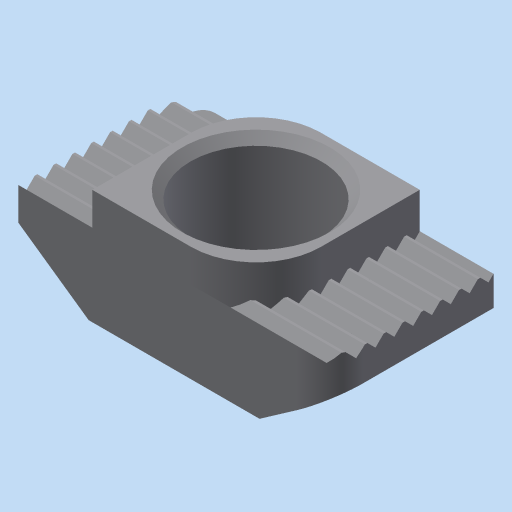
# Autodesk Inventor part: T-NUT - DropIn 4040 SERIES - M8
Saved by Autodesk Inventor 2023.2 (Build 272271000, 271)
## iProperties
Company: TraceParts S.A.
Created: 2023-02-26
Part Number: T-NUT - DropIn 4040 SERIES - M8
Checked By: TraceParts S.A.
Material: Generisch
Catalog Web Link: www.traceparts.com
Document SubType Name: Modeling
Designer: TraceParts
Density: 1 g/cm^3
Appearance: Vorgabe
REFERENCE: 07090-1008017
SUPPLIER: norelem
DESIGN: T-NUT FOR T-SLOT M08 STEEL
TraceParts.PartNumber: 30-06122017-106144
TraceParts.PartTitle: T-NUT FOR T-SLOT M08 STEEL
TraceParts.InstanceId: 30-06122017-1061443DYOD00EO1IYUO4TDSMY561GW
TRACEPARTS: TRACEPARTS
TraceParts.PartLanguage: en
TraceParts.PartVersion: 1.0.7
Author: TraceParts
Autodesk Inventor part; units mm, degrees
ref_plane "YZ Plane" through (0, 0, 0) normal (1, 0, 0) x (0, 1, 0)
ref_plane "XZ Plane" through (0, 0, 0) normal (0, 1, 0) x (-1, 0, 0)
ref_plane "XY Plane" through (0, 0, 0) normal (0, 0, 1) x (1, 0, 0)
sketch "Skizze3" plane through (0, 0, 0) normal (0, 0, 1) x (1, 0, 0)
  line L0 (0, 0) -> (5.215556, 0)
  line L1 (5.215556, 0) -> (9.5, 3)
  line L2 (9.5, 3) -> (9.5, 5)
  line L3 (9.5, 5) -> (0, 5)
  line L4 (0, 6) -> (0, -1) construction
  line L5 (0, 0) -> (-5.215556, 0)
  line L6 (-5.215556, 0) -> (-9.5, 3)
  line L7 (-9.5, 3) -> (-9.5, 5)
  line L8 (-9.5, 5) -> (0, 5)
  dimension "d6" = 9.5
  dimension "d8" = 5
  dimension "d9" = 3
  dimension "d10" = 145
  constraints: 16 end point, 3 symmetric about line, 2 perpendicular, 1 horizontal
  measures "d6" distance between parallel lines of L4 L2
  measures "d8" distance between parallel lines of L0 L3
  measures "d9" distance from line of L0 L1.end
  measures "d10" angle of L0 L1
extrude "Extrusion2" add sketch "Skizze3" along normal mid plane 10
sketch "Skizze4" plane through (-9.5, 5, 5) normal (0, 1, 0) x (1, 0, 0)
  line L0 (0, 10) -> (0, 0)
  line L1 (19, 0) -> (0, 0)
  line L2 (19, 10) -> (19, 0)
  line L3 (0, 10) -> (19, 10)
  circle A0 centre (9.5, 5) radius 4
  line L4 (4.5, 10) -> (14.5, 10)
  line L5 (14.5, 10) -> (14.5, 0)
  line L6 (14.5, 0) -> (4.5, 0)
  line L7 (4.5, 0) -> (4.5, 10)
  line L8 (4.5, 10) -> (14.5, 0) construction
  line L9 (14.5, 10) -> (4.5, 0) construction
  line L10 (0, 10) -> (19, 10)
  arc A1 (8.5, 10) -> (4.5, 6) centre (8.464449, 6.035551) ccw
  arc A2 (10.5, 0) -> (14.5, 4) centre (10.535551, 3.964449) ccw
  point P0 (4.5, 0)
  point P1 (14.5, 0)
  point P2 (4.5, 10)
  point P3 (10.571102, 0)
  point P4 (14.5, 4)
  point P5 (8.428898, 10)
  point P6 (4.5, 6.071102)
  dimension "d13" = 8
  dimension "d14" = 10
  dimension "d15" = 10
  dimension "d37" = 4
  dimension "d38" = 4
  constraints: 12 end point, 4 point on circle, 3 centre point, 3 symmetric about line, 2 midpoint, 2 parallel, 2 point on line, 1 coincident, 1 horizontal, 1 perpendicular, 1 other
  measures "d13" diameter of A0
  measures "d14" distance of L5.end L6.end
  measures "d15" distance of L4.end L5.end
  measures "d37" distance from line of L7 A1.start
  measures "d38" distance from line of L3 A1.end
sketch "Skizze4 outline for Extrusion3" plane through (-9.5, 5, 5) normal (0, 1, 0) x (1, 0, 0)
  arc A0 (10.571102, 0) -> (14.5, 4) centre (10.535551, 3.964449) ccw
  line L0 (4.5, 0) -> (10.571102, 0)
  line L1 (14.5, 4) -> (14.5, 10)
  line L2 (4.5, 6.071102) -> (4.5, 0)
  line L3 (14.5, 10) -> (8.428898, 10)
  arc A1 (8.428898, 10) -> (4.5, 6.071102) centre (8.464449, 6.035551) ccw
  circle A2 centre (9.5, 5) radius 4
extrude "Extrusion3" add sketch "Skizze4 outline for Extrusion3" along normal blind 2 and the other way blind 5 separate body
sketch "Skizze5" plane through (9.5, 3, 5) normal (1, 0, 0) x (0, 0, -1)
  line L0 (10, 2) -> (0, 2)
  line L1 (0, 0) -> (0, 2)
  line L2 (10, 0) -> (0, 0)
  line L3 (10, 2) -> (10, 0)
  line L4 (0, 0) -> (0, 2)
  line L5 (0, 2) -> (0.494975, 1.505025)
  line L6 (0.494975, 1.505025) -> (0.989949, 2)
  line L7 (10, 2) -> (0, 2)
  line L8 (1.15, 2) -> (1.644975, 1.505025)
  line L9 (1.644975, 1.505025) -> (2.139949, 2)
  line L10 (2.3, 2) -> (2.794975, 1.505025)
  line L11 (2.794975, 1.505025) -> (3.289949, 2)
  line L12 (3.45, 2) -> (3.944975, 1.505025)
  line L13 (3.944975, 1.505025) -> (4.439949, 2)
  line L14 (4.6, 2) -> (5.094975, 1.505025)
  line L15 (5.094975, 1.505025) -> (5.589949, 2)
  line L16 (5.75, 2) -> (6.244975, 1.505025)
  line L17 (6.244975, 1.505025) -> (6.739949, 2)
  line L18 (6.9, 2) -> (7.394975, 1.505025)
  line L19 (7.394975, 1.505025) -> (7.889949, 2)
  line L20 (8.05, 2) -> (8.544975, 1.505025)
  line L21 (8.544975, 1.505025) -> (9.039949, 2)
  line L22 (9.2, 2) -> (9.694975, 1.505025)
  line L23 (9.694975, 1.505025) -> (10.189949, 2)
  point P0 (5, -3)
  point P1 (10, 1.810051)
  dimension "d21" = 0.7
  dimension "d24" = 1.15
  constraints: 36 end point, 2 perpendicular, 1 horizontal, 1 point on line, 40 other
  measures "d21" distance of L0.end L5.end
  measures "d24" distance of L0.end L8.start
extrude "Extrusion4" cut sketch "Skizze5" against normal up to surface (19 mm away) contours L3 L23 L22 L0 | L21 L20 L0 | L19 L18 L0 | L0 L6 L5 | L17 L16 L0 | L0 L9 L8 | L15 L14 L0 | L0 L11 L10 | L13 L12 L0 bodies 1
extrude "Extrusion5" cut sketch "Skizze4" against normal blind 10 contours A0 bodies 1
chamfer "Fase2" distance 0.5 angle 45 1 edges at (-4, 7, 0)
combine bodies "Kombinieren1" operation type add bodies to combine 1 2
fillet "Rundung1" radius 2 2 edges at (9.5, 4, 5) (-9.5, 3.905, -5)
equation "\"d38\" = d37"
